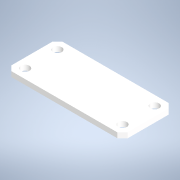
# Autodesk Inventor part: Platina
Saved by Autodesk Inventor 2022 (Build 260153000, 153)
## iProperties
Created: 2021-10-23
Part Number: Platina
Material: PET Plastic
Document SubType Name: Modeling
Designer: juanp
Density: 1.541 g/cm^3
Appearance: Polycarbonate - Clear
Author: juanp
Autodesk Inventor part; units mm, degrees
ref_plane "YZ Plane" through (0, 0, 0) normal (1, 0, 0) x (0, 1, 0)
ref_plane "XZ Plane" through (0, 0, 0) normal (0, 1, 0) x (-1, 0, 0)
ref_plane "XY Plane" through (0, 0, 0) normal (0, 0, 1) x (1, 0, 0)
sketch "Sketch1" plane through (0, 0, 0) normal (0, 1, 0) x (-1, 0, 0)
  line L0 (28.75, 9.525) -> (-28.75, 9.525) construction
  line L1 (-28.75, 9.525) -> (-28.75, -9.525) construction
  line L2 (-28.75, -9.525) -> (28.75, -9.525) construction
  line L3 (28.75, -9.525) -> (28.75, 9.525) construction
  line L4 (28.75, 9.525) -> (-28.75, -9.525) construction
  line L5 (-28.75, 9.525) -> (28.75, -9.525) construction
  circle A0 centre (28.75, 9.525) radius 2.55
  circle A1 centre (28.75, -9.525) radius 2.55
  circle A2 centre (-28.75, 9.525) radius 2.55
  circle A3 centre (-28.75, -9.525) radius 2.55
  line L6 (34.3, 15.075) -> (-34.3, 15.075)
  line L7 (-34.3, 15.075) -> (-34.3, -15.075)
  line L8 (-34.3, -15.075) -> (34.3, -15.075)
  line L9 (34.3, -15.075) -> (34.3, 15.075)
  line L10 (34.3, 15.075) -> (-34.3, -15.075) construction
  line L11 (-34.3, 15.075) -> (34.3, -15.075) construction
  point P0 (0, 0)
  dimension "d0" = 19.05
  dimension "d1" = 57.5
  dimension "d2" = 5.1
  dimension "d3" = 3
  dimension "d4" = 3
  constraints: 24 end point, 4 centre point, 4 coincident, 4 midpoint, 4 parallel, 3 equal radius, 2 horizontal, 2 perpendicular
  measures "d0" distance of L2.end L0.start
  measures "d1" distance of L1.end L2.end
  measures "d2" diameter of A1
  measures "d3" distance edge to line of A3 L7
  measures "d4" distance edge to line of A3 L8
extrude "Extrusion1" add sketch "Sketch1" along normal blind 3
chamfer "Chamfer1" distance 3 angle 45 4 edges at (-34.3, 1.5, 15.075) (-34.3, 1.5, -15.075) (34.3, 1.5, -15.075) (34.3, 1.5, 15.075)
body "Solid1"
